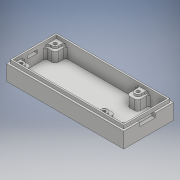
# Autodesk Inventor part: bottom
Saved by Autodesk Inventor 2018 (Build 220112000, 112)
## iProperties
Created: 2018-01-10
Part Number: bottom
Material: Generic
Document SubType Name: Modeling
Designer: gregg
Density: 1 g/cm^3
Appearance: Default
Author: gregg
Autodesk Inventor part; units mm, degrees
ref_plane "YZ Plane" through (0, 0, 0) normal (1, 0, 0) x (0, 1, 0)
ref_plane "XZ Plane" through (0, 0, 0) normal (0, 1, 0) x (-1, 0, 0)
ref_plane "XY Plane" through (0, 0, 0) normal (0, 0, 1) x (1, 0, 0)
sketch "Sketch1" plane through (0, 0, 0) normal (0, 0, 1) x (1, 0, 0)
  line L0 (0, 0) -> (100, 0)
  line L1 (100, 0) -> (100, 39)
  line L2 (100, 39) -> (0, 39)
  line L3 (0, 39) -> (0, 0)
  dimension "d46" = 39
  dimension "d47" = 100
  constraints: 8 end point, 2 parallel, 1 horizontal, 1 perpendicular
  measures "d46" distance between parallel lines of L0 L2
  measures "d47" distance between parallel lines of L1 L3
extrude "bottom" add sketch "Sketch1" along normal blind 3
sketch "Sketch5" plane through (0, 0, 0) normal (0, 0, -1) x (-1, 0, 0)
  line L0 (0, 0) -> (-100, 0) projected
  line L1 (0, 39) -> (0, 0) projected
  line L2 (-100, 39) -> (0, 39) projected
  line L3 (-100, 0) -> (-100, 39) projected
  line L4 (3, 42) -> (3, -3)
  line L5 (3, -3) -> (-103, -3)
  line L6 (-103, -3) -> (-103, 42)
  line L7 (-103, 42) -> (3, 42)
  dimension "d30" = 3
  constraints: 8 end point, 3 other
  measures "d30" distance between parallel lines of L2 L7
extrude "walls" add sketch "Sketch5" against normal blind 14
sketch "holes" plane through (0, 0, 3) normal (0, 0, 1) x (1, 0, 0)
  line L0 (0, 0) -> (100, 0) projected
  line L1 (100, 0) -> (100, 39) projected
  line L2 (100, 39) -> (0, 39) projected
  line L3 (0, 39) -> (0, 0) projected
  circle A0 centre (3.5, 34.5) radius 1.55 construction
  circle A1 centre (78.5, 34.5) radius 1.55 construction
  circle A2 centre (78.5, 3.5) radius 1.55 construction
  circle A3 centre (3.5, 3.5) radius 1.55 construction
  line L4 (3.5, 34.5) -> (3.5, 3.5) construction
  line L5 (3.5, 3.5) -> (78.5, 3.5) construction
  line L6 (78.5, 3.5) -> (78.5, 34.5) construction
  line L7 (78.5, 34.5) -> (3.5, 34.5) construction
  dimension "d33" = 3.1
  dimension "d34" = 75
  dimension "d35" = 31
  dimension "d58" = 3.5
  dimension "d59" = 3.5
  constraints: 8 end point, 4 centre point, 3 equal radius, 2 horizontal, 2 vertical
  measures "d33" diameter of A0
  measures "d34" distance of L6.end L4.start
  measures "d35" distance of L4.end L4.start
  measures "d58" distance from line of L4.end L3
  measures "d59" distance from line of L0 L4.end
sketch "Sketch8" plane through (103, -3, 0) normal (1, 0, 0) x (0, 0, -1)
  line L0 (-10.5, 14.297) -> (-14, 14.297)
  line L1 (-14, 14.297) -> (-14, 28.297)
  line L2 (-14, 28.297) -> (-10.5, 28.297)
  line L3 (-10.5, 28.297) -> (-10.5, 14.297)
  line L4 (-14, 0) -> (-14, 45) projected
  line L5 (-14, 28.297) -> (-10.5, 14.297) construction
  line L6 (-10.5, 28.297) -> (-14, 14.297) construction
  point P0 (0, 3)
  point P1 (-3, 37.5)
  point P2 (-3, 6.5)
  point P3 (-12.25, 21.297)
  dimension "d50" = 3.5
  dimension "d108" = 14.797
  dimension "d109" = 14
  constraints: 12 end point, 2 parallel, 1 horizontal, 1 midpoint, 1 perpendicular, 1 point on line
  measures "d50" distance of L1.end L2.end
  measures "d108" vertical distance of point (-3, 6.5) point (-12.25, 21.297)
  measures "d109" distance of L0.end L1.end
extrude "tip" cut sketch "Sketch8" against normal up to surface (3 mm away)
sketch "Sketch9" plane through (-3, -3, 0) normal (-1, 0, 0) x (0, 0, 1)
  line L0 (14, 16.412) -> (11, 16.412)
  line L1 (11, 16.412) -> (11, 24.912)
  line L2 (11, 24.912) -> (14, 24.912)
  line L3 (14, 24.912) -> (14, 16.412)
  line L4 (14, 45) -> (14, 0) projected
  line L5 (14, 25.5761) -> (11, 16.412) construction
  line L6 (14, 16.412) -> (11, 24.912) construction
  point P0 (0, 3)
  point P1 (3, 6.5)
  point P2 (3, 37.5)
  point P3 (3, 37.5)
  point P4 (3, 37.5)
  point P5 (12.5, 20.662)
  dimension "d53" = 3
  dimension "d110" = 14.162
  dimension "d111" = 8.5
  constraints: 12 end point, 2 parallel, 2 point on line, 1 horizontal, 1 midpoint, 1 perpendicular
  measures "d53" distance of L0.start L0.end
  measures "d110" vertical distance of point (3, 6.5) point (12.5, 20.662)
  measures "d111" distance of L2.end L0.start
extrude "uart" cut sketch "Sketch9" against normal up to surface (3 mm away)
sketch "Sketch7" plane through (0, 0, 3) normal (0, 0, 1) x (1, 0, 0)
  circle A0 centre (3.5, 34.5) radius 1.55 construction
  circle A1 centre (3.5, 3.5) radius 1.55 construction
  circle A2 centre (78.5, 3.5) radius 1.55 construction
  circle A3 centre (78.5, 34.5) radius 1.55 construction
  line L0 (0, 39) -> (0, 0) projected
  line L1 (2, 29.5) -> (8.5, 29.5)
  line L2 (8.5, 29.5) -> (8.5, 37)
  line L3 (100, 39) -> (0, 39) projected
  arc A4 (10.5, 39) -> (8.5, 37) centre (10.5, 37) ccw
  line L4 (0, 39) -> (100, 39) projected
  arc A5 (5.4, 29.5) -> (8.5, 32.6) centre (5.4, 32.6) ccw
  arc A6 (2, 29.5) -> (0, 27.5) centre (2, 27.5) ccw
  line L5 (0, 0) -> (0, 39) projected
  line L6 (1.7924, 37.3805) -> (5.1408, 37.4191)
  line L7 (5.1408, 37.4191) -> (6.8484, 34.5385)
  line L8 (6.8484, 34.5385) -> (5.2076, 31.6195)
  line L9 (5.2076, 31.6195) -> (1.8592, 31.5809)
  line L10 (1.8592, 31.5809) -> (0.1516, 34.4615)
  line L11 (0.1516, 34.4615) -> (1.7924, 37.3805)
  line L12 (100, 0) -> (0, 0) projected
  line L13 (0, 0) -> (0, 10.5)
  arc A7 (0, 10.5) -> (2, 8.5) centre (2, 10.5) ccw
  line L14 (2, 8.5) -> (5.4, 8.5)
  arc A8 (8.5, 5.4) -> (5.4, 8.5) centre (5.4, 5.4) ccw
  line L15 (8.5, 5.4) -> (8.5, 2)
  arc A9 (8.5, 2) -> (10.5, 0) centre (10.5, 2) ccw
  line L16 (10.5, 0) -> (0, 0)
  line L17 (85.5, 39) -> (71.5, 39)
  arc A10 (73.5, 37) -> (71.5, 39) centre (71.5, 37) ccw
  line L18 (73.5, 37) -> (73.5, 32.0359)
  line L19 (83.5, 32.0359) -> (83.5, 37)
  arc A11 (85.5, 39) -> (83.5, 37) centre (85.5, 37) ccw
  line L20 (71.5, 0) -> (85.5, 0)
  line L21 (0, 0) -> (100, 0) projected
  arc A12 (83.5, 2) -> (85.5, 0) centre (85.5, 2) ccw
  line L22 (83.5, 2) -> (83.5, 5.9641)
  line L23 (73.5, 5.9641) -> (73.5, 2)
  arc A13 (71.5, 0) -> (73.5, 2) centre (71.5, 2) ccw
  arc A14 (76.5, 8.9641) -> (73.5, 5.9641) centre (76.5, 5.9641) ccw
  line L24 (76.5, 8.9641) -> (80.5, 8.9641)
  arc A15 (83.5, 5.9641) -> (80.5, 8.9641) centre (80.5, 5.9641) ccw
  arc A16 (73.5, 32.0359) -> (76.5, 29.0359) centre (76.5, 32.0359) ccw
  arc A17 (80.5, 29.0359) -> (83.5, 32.0359) centre (80.5, 32.0359) ccw
  line L25 (76.5, 29.0359) -> (80.5, 29.0359)
  line L26 (75.5, 1.7679) -> (75.5, 5.2321) construction
  line L27 (75.5, 5.2321) -> (78.5, 6.9641) construction
  line L28 (78.5, 6.9641) -> (81.5, 5.2321) construction
  line L29 (81.5, 5.2321) -> (81.5, 1.7679) construction
  line L30 (81.5, 1.7679) -> (78.5, 0.0359) construction
  line L31 (78.5, 0.0359) -> (75.5, 1.7679) construction
  line L32 (78.5, 31.0359) -> (75.5, 32.7679) construction
  line L33 (75.5, 32.7679) -> (75.5, 36.2321) construction
  line L34 (75.5, 36.2321) -> (78.5, 37.9641) construction
  line L35 (78.5, 37.9641) -> (81.5, 36.2321) construction
  line L36 (81.5, 36.2321) -> (81.5, 32.7679) construction
  line L37 (81.5, 32.7679) -> (78.5, 31.0359) construction
  line L38 (78.5, 34.5) -> (73.5, 34.5) construction
  line L39 (78.5, 34.5) -> (83.5, 34.5) construction
  point P0 (78.5, 29.5)
  point P1 (78.5, 29.5)
  point P2 (78.5, 18.273)
  point P3 (78.5, 18.273)
  dimension "d38" = 5
  dimension "d39" = 5
  dimension "d40" = 2
  dimension "d41" = 3.1
  dimension "d42" = 2
  dimension "d60" = 5.8
  dimension "d77" = 5
  dimension "d78" = 5
  dimension "d79" = 3.1
  dimension "d87" = 6
  dimension "d88" = 10
  dimension "d89" = 2
  dimension "d90" = 3
  dimension "d91" = 6
  dimension "d92" = 2
  constraints: 68 end point, 28 point on circle, 28 tangent, 14 centre point, 12 point on line, 9 equal radius, 7 vertical, 5 coincident, 5 horizontal, 3 collinear, 3 perpendicular, 43 other
  measures "d38" distance from line of L2 A0.centre
  measures "d39" distance from line of L1 A0.centre
  measures "d40" radius of A4
  measures "d41" radius of A5
  measures "d42" radius of A6
  measures "d60" distance between parallel lines of L9 L6
  measures "d77" distance from line of L14 A1.centre
  measures "d78" distance from line of L15 A1.centre
  measures "d79" radius of A8
  measures "d87" distance between parallel lines of L26 L29
  measures "d88" distance between parallel lines of L22 L23
  measures "d89" distance from line of L24 L27.end
  measures "d90" radius of A15
  measures "d91" distance between parallel lines of L36 L33
  measures "d92" distance from line of L25 L32.start
extrude "standoffs" add sketch "Sketch7" along normal blind 9 contours L3 A4 L2 A5 L1 A6 L0 | L3 A11 L19 A17 L25 A16 L18 A10 | A13 L23 A14 L24 A15 L22 A12 L12 | A7 L14 A8 L15 A9 L12 L0 | L6 L7 L8 L9 L10 L11
sketch "Sketch10" plane through (0, 0, 12) normal (0, 0, 1) x (1, 0, 0)
  line L0 (2, 31.5) -> (3.4, 31.5)
  arc A0 (3.4, 31.5) -> (6.5, 34.6) centre (3.4, 34.6) ccw
  line L1 (6.5, 34.6) -> (6.5, 37)
  arc A1 (8.5, 39) -> (6.5, 37) centre (8.5, 37) ccw
  line L2 (8.5, 39) -> (0, 39)
  line L3 (0, 39) -> (0, 29.5)
  arc A2 (2, 29.5) -> (0, 27.5) centre (2, 27.5) ccw projected
  line L4 (2, 29.5) -> (5.4, 29.5) projected
  arc A3 (5.4, 29.5) -> (8.5, 32.6) centre (5.4, 32.6) ccw projected
  line L5 (8.5, 32.6) -> (8.5, 37) projected
  arc A4 (10.5, 39) -> (8.5, 37) centre (10.5, 37) ccw projected
  line L6 (0, 39) -> (10.5, 39) projected
  line L7 (0, 27.5) -> (0, 39) projected
  arc A5 (2, 31.5) -> (0, 29.5) centre (2, 29.5) ccw
  line L8 (3.5, 34.5) -> (3.5, 3.5) construction
  line L9 (78.5, 34.5) -> (3.5, 34.5) construction
  line L10 (0, 0) -> (0, 8.5)
  arc A6 (0, 8.5) -> (2, 6.5) centre (2, 8.5) ccw
  line L11 (2, 6.5) -> (3.4, 6.5)
  arc A7 (6.5, 3.4) -> (3.4, 6.5) centre (3.4, 3.4) ccw
  line L12 (6.5, 3.4) -> (6.5, 2)
  arc A8 (6.5, 2) -> (8.5, 0) centre (8.5, 2) ccw
  line L13 (8.5, 0) -> (0, 0)
  line L14 (100, 0) -> (0, 0) projected
  line L15 (78.5, 3.5) -> (78.5, 34.5) construction
  line L16 (3.5, 3.5) -> (78.5, 3.5) construction
  line L17 (71.5, 39) -> (85.5, 39) projected
  line L18 (73.5, 39) -> (83.5, 39)
  arc A9 (83.5, 39) -> (81.5, 37) centre (83.5, 37) ccw
  line L19 (81.5, 37) -> (81.5, 34.5)
  line L20 (75.5, 34.5) -> (75.5, 37)
  arc A10 (75.5, 37) -> (73.5, 39) centre (73.5, 37) ccw
  line L21 (0, 39) -> (100, 39) projected
  arc A11 (75.5, 34.5) -> (81.5, 34.5) centre (78.5, 34.5) ccw
  arc A12 (81.5, 3.5) -> (75.5, 3.5) centre (78.5, 3.5) ccw
  line L22 (81.5, 3.5) -> (81.5, 2)
  arc A13 (81.5, 2) -> (83.5, 0) centre (83.5, 2) ccw
  line L23 (83.5, 0) -> (73.5, 0)
  arc A14 (73.5, 0) -> (75.5, 2) centre (73.5, 2) ccw
  line L24 (75.5, 2) -> (75.5, 3.5)
  dimension "d61" = 3
  dimension "d62" = 3
  dimension "d63" = 2
  dimension "d64" = 3.1
  dimension "d65" = 2
  dimension "d80" = 3
  dimension "d81" = 3
  dimension "d96" = 6
  dimension "d97" = 6
  constraints: 28 end point, 25 tangent, 24 point on circle, 12 centre point, 7 equal radius, 6 point on line, 6 vertical, 3 perpendicular, 2 coincident, 1 horizontal
  measures "d61" distance from line of L0 L8.start
  measures "d62" distance from line of L1 L8.start
  measures "d63" radius of A1
  measures "d64" radius of A0
  measures "d65" radius of A5
  measures "d80" distance from line of L11 L8.end
  measures "d81" distance from line of L12 L8.end
  measures "d96" diameter of A11
  measures "d97" diameter of A12
extrude "finalStandoff" add sketch "Sketch10" along normal up to surface (2 mm away) contours A5 L3 L2 A1 L1 A0 L0 | L17 A9 L19 A11 L20 A10 | A14 L24 A12 L22 A13 L14 | L10 A6 L11 A7 L12 A8 L13
sketch "Sketch11" plane through (0, 0, 0) normal (0, 0, -1) x (-1, 0, 0)
  line L0 (-78.5, 34.5) -> (-3.5, 34.5) construction
  line L1 (-3.5, 34.5) -> (-3.5, 3.5) construction
  line L2 (-2.6034, 31.1539) -> (-5.9495, 32.0505)
  line L3 (-5.9495, 32.0505) -> (-6.8461, 35.3966)
  line L4 (-6.8461, 35.3966) -> (-4.3966, 37.8461)
  line L5 (-4.3966, 37.8461) -> (-1.0505, 36.9495)
  line L6 (-1.0505, 36.9495) -> (-0.1539, 33.6034)
  line L7 (-0.1539, 33.6034) -> (-2.6034, 31.1539)
  line L8 (-5.9495, 32.0505) -> (-3.5, 34.5) construction
  line L9 (-5.9495, 5.9495) -> (-2.6034, 6.8461)
  line L10 (-2.6034, 6.8461) -> (-0.1539, 4.3966)
  line L11 (-0.1539, 4.3966) -> (-1.0505, 1.0505)
  line L12 (-1.0505, 1.0505) -> (-4.3966, 0.1539)
  line L13 (-4.3966, 0.1539) -> (-6.8461, 2.6034)
  line L14 (-6.8461, 2.6034) -> (-5.9495, 5.9495)
  line L15 (-5.9495, 32.0505) -> (-5.9495, 5.9495) construction
  line L16 (-78.5, 3.5) -> (-78.5, 34.5) construction
  line L17 (-3.5, 3.5) -> (-78.5, 3.5) construction
  line L18 (-78.5, 31.0359) -> (-81.5, 32.7679)
  line L19 (-81.5, 32.7679) -> (-81.5, 36.2321)
  line L20 (-81.5, 36.2321) -> (-78.5, 37.9641)
  line L21 (-78.5, 37.9641) -> (-75.5, 36.2321)
  line L22 (-75.5, 36.2321) -> (-75.5, 32.7679)
  line L23 (-75.5, 32.7679) -> (-78.5, 31.0359)
  line L24 (-75.5, 5.2321) -> (-75.5, 1.7679)
  line L25 (-75.5, 1.7679) -> (-78.5, 0.0359)
  line L26 (-78.5, 0.0359) -> (-81.5, 1.7679)
  line L27 (-81.5, 1.7679) -> (-81.5, 5.2321)
  line L28 (-81.5, 5.2321) -> (-78.5, 6.9641)
  line L29 (-78.5, 6.9641) -> (-75.5, 5.2321)
  point P0 (0, 0)
  dimension "d68" = 6
  dimension "d69" = 45
  constraints: 52 end point, 4 coincident, 3 equal length, 3 vertical, 52 other
  measures "d68" distance between parallel lines of L4 L7
  measures "d69" angle of L0 L8
extrude "forNuts" cut sketch "Sketch11" against normal up to surface (12 mm away)
sketch "Sketch13" plane through (0, 0, 0) normal (0, 0, -1) x (-1, 0, 0)
  circle A0 centre (-3.5, 34.5) radius 1.55
  circle A1 centre (-3.5, 3.5) radius 1.55 projected
  circle A2 centre (-78.5, 34.5) radius 1.55 projected
  circle A3 centre (-78.5, 3.5) radius 1.55 projected
  point P0 (0, 0)
  dimension "d74" = 3.1
  constraints: 1 centre point, 1 coincident
  measures "d74" diameter of A0
extrude "mountHoles" cut sketch "Sketch13" along normal through all both and the other way through all
sketch "Sketch12" plane through (3.4, 31.5, 12) normal (0, 0, -1) x (-1, 0, 0)
  line L0 (-3.4461, 3.8966) -> (-0.9966, 6.3461) projected
  line L1 (-0.9966, 6.3461) -> (2.3495, 5.4495) projected
  line L2 (2.3495, 5.4495) -> (3.2461, 2.1034) projected
  line L3 (3.2461, 2.1034) -> (0.7966, -0.3461) projected
  line L4 (0.7966, -0.3461) -> (-2.5495, 0.5505) projected
  line L5 (-2.5495, 0.5505) -> (-3.4461, 3.8966) projected
  line L6 (2.3495, -30.4495) -> (-0.9966, -31.3461) projected
  line L7 (-0.9966, -31.3461) -> (-3.4461, -28.8966) projected
  line L8 (-3.4461, -28.8966) -> (-2.5495, -25.5505) projected
  line L9 (-2.5495, -25.5505) -> (0.7966, -24.6539) projected
  line L10 (0.7966, -24.6539) -> (3.2461, -27.1034) projected
  line L11 (3.2461, -27.1034) -> (2.3495, -30.4495) projected
  line L12 (6.4, 10.5) -> (6.4, -34.5) projected
  line L13 (-99.6, 10.5) -> (6.4, 10.5) projected
  line L14 (-99.6, -34.5) -> (-99.6, 10.5) projected
  line L15 (6.4, -34.5) -> (-99.6, -34.5) projected
  line L16 (-78.1, 4.7321) -> (-75.1, 6.4641) projected
  line L17 (-75.1, 6.4641) -> (-72.1, 4.7321) projected
  line L18 (-72.1, 4.7321) -> (-72.1, 1.2679) projected
  line L19 (-72.1, 1.2679) -> (-75.1, -0.4641) projected
  line L20 (-75.1, -0.4641) -> (-78.1, 1.2679) projected
  line L21 (-78.1, 1.2679) -> (-78.1, 4.7321) projected
  line L22 (-78.1, -29.7321) -> (-78.1, -26.2679) projected
  line L23 (-78.1, -26.2679) -> (-75.1, -24.5359) projected
  line L24 (-75.1, -24.5359) -> (-72.1, -26.2679) projected
  line L25 (-72.1, -26.2679) -> (-72.1, -29.7321) projected
  line L26 (-72.1, -29.7321) -> (-75.1, -31.4641) projected
  line L27 (-75.1, -31.4641) -> (-78.1, -29.7321) projected
  line L28 (3.2461, -27.1034) -> (2.3495, -30.4495) projected
  line L29 (2.3495, -30.4495) -> (-0.9966, -31.3461) projected
  line L30 (-0.9966, -31.3461) -> (-3.4461, -28.8966) projected
  line L31 (-3.4461, -28.8966) -> (-2.5495, -25.5505) projected
  line L32 (-2.5495, -25.5505) -> (0.7966, -24.6539) projected
  line L33 (0.7966, -24.6539) -> (3.2461, -27.1034) projected
  line L34 (-0.9966, 6.3461) -> (2.3495, 5.4495) projected
  line L35 (2.3495, 5.4495) -> (3.2461, 2.1034) projected
  line L36 (3.2461, 2.1034) -> (0.7966, -0.3461) projected
  line L37 (0.7966, -0.3461) -> (-2.5495, 0.5505) projected
  line L38 (-2.5495, 0.5505) -> (-3.4461, 3.8966) projected
  line L39 (-3.4461, 3.8966) -> (-0.9966, 6.3461) projected
  line L40 (6.4, 10.5) -> (6.4, -34.5) projected
  line L41 (-99.6, 10.5) -> (6.4, 10.5) projected
  line L42 (-99.6, -34.5) -> (-99.6, 10.5) projected
  line L43 (6.4, -34.5) -> (-99.6, -34.5) projected
extrude "fillBeforeHoles" add sketch "Sketch12" along normal blind 0.6 contours L0 L1 L2 L3 L4 L5 | L6 L7 L8 L9 L10 L11 | L16 L17 L18 L19 L20 L21 | L22 L23 L24 L25 L26 L27
sketch "Sketch14" plane through (0, 0, 3) normal (0, 0, 1) x (1, 0, 0)
  line L0 (21.673, 4.45) -> (35.673, 4.45)
  line L1 (35.673, 4.45) -> (35.673, 0.95)
  line L2 (35.673, 0.95) -> (21.673, 0.95)
  line L3 (21.673, 0.95) -> (21.673, 4.45)
  line L4 (3.5, 34.5) -> (3.5, 3.5) construction
  line L5 (3.5, 3.5) -> (78.5, 3.5) construction
  line L6 (21.673, 4.45) -> (35.673, 0.95) construction
  line L7 (35.673, 4.45) -> (21.673, 0.95) construction
  point P0 (0, 0)
  point P1 (28.673, 2.7)
  dimension "d112" = 25.173
  dimension "d113" = 0.8
  dimension "d114" = 3.5
  dimension "d115" = 14
  constraints: 12 end point, 2 parallel, 1 horizontal, 1 midpoint, 1 perpendicular
  measures "d112" horizontal distance of point (28.673, 2.7) L4.end
  measures "d113" vertical distance of point (28.673, 2.7) L4.end
  measures "d114" distance of L2.end L0.start
  measures "d115" distance of L1.end L2.end
extrude "jtag" cut sketch "Sketch14" along normal through all both and the other way through all
sketch "Sketch21" plane through (0, 0, 3) normal (0, 0, 1) x (1, 0, 0)
  circle A0 centre (91.75, 6.5) radius 7
  line L0 (83.5, 2) -> (83.5, 5.9641) projected
  line L1 (83.5, 6.5) -> (91.75, 6.5) construction
  line L2 (91.75, 6.5) -> (100, 6.5) construction
  line L3 (100, 0) -> (83.5, 0) projected
  line L4 (100, 11.297) -> (100, 0) projected
  arc A1 (83.5, 5.9641) -> (80.5, 8.9641) centre (80.5, 5.9641) ccw projected
  arc A2 (80.5, 8.9641) -> (86.8946, 11.5424) centre (80.5, 18.1833) ccw
  line L5 (80.5, 8.9641) -> (76.5, 8.9641) projected
  line L6 (100, 11.297) -> (100, 25.297) projected
  arc A3 (97.4895, 10.5073) -> (100, 11.297) centre (98.6205, 11.297) ccw
  arc A4 (83.5, 2) -> (85.5, 0) centre (85.5, 2) ccw projected
  line L7 (85.5, 0) -> (89.1519, 0)
  line L8 (85.5, 0) -> (100, 0) projected
  line L9 (94.3481, 0) -> (100, 0)
  point P0 (0, 0)
  dimension "d134" = 14
  dimension "d135" = 6.5
  constraints: 8 end point, 8 point on circle, 4 point on line, 4 tangent, 3 centre point, 2 collinear, 1 horizontal, 1 perpendicular
  measures "d134" diameter of A0
  measures "d135" distance from line of L3 L1.end
extrude "Extrusion21" add sketch "Sketch21" along normal blind 2.7
sketch "Sketch15" plane through (0, 0, 3) normal (0, 0, 1) x (1, 0, 0)
  circle A0 centre (91.75, 6.5) radius 4
  line L0 (35.673, 4.45) -> (35.673, 0.95) construction
  line L1 (35.673, 0.95) -> (21.673, 0.95) construction
  line L2 (21.673, 0.95) -> (21.673, 4.45) construction
  line L3 (21.673, 4.45) -> (35.673, 4.45) construction
  arc A1 (71.5, 0) -> (73.5, 2) centre (71.5, 2) ccw construction
  line L4 (73.5, 2) -> (73.5, 5.9641) construction
  arc A2 (76.5, 8.9641) -> (73.5, 5.9641) centre (76.5, 5.9641) ccw construction
  line L5 (76.5, 8.9641) -> (80.5, 8.9641) construction
  line L6 (100, 11.297) -> (100, 39) construction
  line L7 (100, 39) -> (85.5, 39) construction
  arc A3 (85.5, 39) -> (83.5, 37) centre (85.5, 37) ccw construction
  line L8 (83.5, 37) -> (83.5, 32.0359) construction
  arc A4 (80.5, 29.0359) -> (83.5, 32.0359) centre (80.5, 32.0359) ccw construction
  line L9 (80.5, 29.0359) -> (76.5, 29.0359) construction
  arc A5 (73.5, 32.0359) -> (76.5, 29.0359) centre (76.5, 32.0359) ccw construction
  line L10 (73.5, 32.0359) -> (73.5, 37) construction
  arc A6 (73.5, 37) -> (71.5, 39) centre (71.5, 37) ccw construction
  line L11 (71.5, 39) -> (10.5, 39) construction
  arc A7 (10.5, 39) -> (8.5, 37) centre (10.5, 37) ccw construction
  line L12 (8.5, 37) -> (8.5, 32.6) construction
  arc A8 (5.4, 29.5) -> (8.5, 32.6) centre (5.4, 32.6) ccw construction
  line L13 (5.4, 29.5) -> (2, 29.5) construction
  arc A9 (2, 29.5) -> (0, 27.5) centre (2, 27.5) ccw construction
  line L14 (0, 27.5) -> (0, 10.5) construction
  arc A10 (0, 10.5) -> (2, 8.5) centre (2, 10.5) ccw construction
  line L15 (2, 8.5) -> (5.4, 8.5) construction
  arc A11 (8.5, 5.4) -> (5.4, 8.5) centre (5.4, 5.4) ccw construction
  line L16 (8.5, 5.4) -> (8.5, 2) construction
  arc A12 (8.5, 2) -> (10.5, 0) centre (10.5, 2) ccw construction
  line L17 (10.5, 0) -> (71.5, 0) construction
  line L18 (91.75, 6.5) -> (83.5, 6.5) construction
  line L19 (91.75, 6.5) -> (100, 6.5) construction
  circle A13 centre (91.75, 6.5) radius 4.5 construction
  line L20 (84.8812, 11) -> (104.9849, 11) construction
  circle A14 centre (91.75, 6.5) radius 5.5 construction
  arc A15 (97.4895, 10.5073) -> (86.8946, 11.5424) centre (91.75, 6.5) ccw projected
  arc A16 (80.5, 8.9641) -> (86.8946, 11.5424) centre (80.5, 18.1833) ccw projected
  arc A17 (97.4895, 10.5073) -> (100, 11.297) centre (98.6205, 11.297) ccw projected
  point P0 (0, 0)
  dimension "d104" = 8
  dimension "d116" = 9
  dimension "d117" = 11
  constraints: 6 end point, 3 centre point, 2 coincident, 2 horizontal, 1 collinear, 1 point on line, 1 tangent
  measures "d104" diameter of A0
  measures "d116" diameter of A13
  measures "d117" diameter of A14
extrude "power" cut sketch "Sketch15" along normal through all both and the other way through all
sketch "Sketch16" plane through (0, 0, 0) normal (0, 0, -1) x (-1, 0, 0)
  circle A0 centre (-91.75, 6.5) radius 4 projected
  line L0 (-88.7478, 11.7) -> (-85.7456, 6.5)
  line L1 (-85.7456, 6.5) -> (-88.7478, 1.3)
  line L2 (-88.7478, 1.3) -> (-94.7522, 1.3)
  line L3 (-94.7522, 1.3) -> (-97.7544, 6.5)
  line L4 (-97.7544, 6.5) -> (-94.7522, 11.7)
  line L5 (-94.7522, 11.7) -> (-88.7478, 11.7)
  point P0 (0, 0)
  dimension "d118" = 10.4
  constraints: 12 end point, 1 coincident, 1 horizontal, 13 other
  measures "d118" distance between parallel lines of L2 L5
extrude "powerNut" cut sketch "Sketch16" against normal blind 3.1
sketch "Sketch17" plane through (0, 0, 3.1) normal (0, 0, -1) x (-1, 0, 0)
  line L0 (-88.7478, 11.7) -> (-85.7456, 6.5) projected
  line L1 (-94.7522, 11.7) -> (-88.7478, 11.7) projected
  line L2 (-97.7544, 6.5) -> (-94.7522, 11.7) projected
  line L3 (-94.7522, 1.3) -> (-97.7544, 6.5) projected
  line L4 (-88.7478, 1.3) -> (-94.7522, 1.3) projected
  line L5 (-85.7456, 6.5) -> (-88.7478, 1.3) projected
  point P0 (0, 0)
extrude "fillBeforePowerNut" add sketch "Sketch17" along normal blind 0.6
sketch "Sketch18" plane through (0, 0, 0) normal (0, 0, -1) x (-1, 0, 0)
  line L0 (-8.5363, 30.1182) -> (10.4943, 30.1182) construction
  line L1 (10.4943, 30.1182) -> (10.4943, 25.4403) construction
  line L2 (10.4943, 25.4403) -> (-8.5363, 25.4403) construction
  line L3 (-8.5363, 25.4403) -> (-8.5363, 30.1182) construction
  line L4 (-9.0093, 21.9531) -> (10.0213, 21.9531) construction
  line L5 (10.0213, 21.9531) -> (10.0213, 17.2752) construction
  line L6 (10.0213, 17.2752) -> (-9.0093, 17.2752) construction
  line L7 (-9.0093, 17.2752) -> (-9.0093, 21.9531) construction
  line L8 (-14.7037, 9.2364) -> (-14.7037, 13.9143) construction
  line L9 (-14.7037, 13.9143) -> (4.3268, 13.9143) construction
  line L10 (4.3268, 13.9143) -> (4.3268, 9.2364) construction
  line L11 (4.3268, 9.2364) -> (-14.7037, 9.2364) construction
  line L12 (-45.6184, 12.2142) -> (-26.5878, 12.2142) construction
  line L13 (-26.5878, 12.2142) -> (-26.5878, 7.5363) construction
  line L14 (-26.5878, 7.5363) -> (-45.6184, 7.5363) construction
  line L15 (-45.6184, 7.5363) -> (-45.6184, 12.2142) construction
  line L16 (-40.2506, 5.3058) -> (-21.22, 5.3058) construction
  line L17 (-21.22, 5.3058) -> (-21.22, 0.6279) construction
  line L18 (-21.22, 0.6279) -> (-40.2506, 0.6279) construction
  line L19 (-40.2506, 0.6279) -> (-40.2506, 5.3058) construction
  line L20 (-101.9782, 14.4275) -> (-101.9782, 19.1054) construction
  line L21 (-101.9782, 19.1054) -> (-61.9534, 19.1054) construction
  line L22 (-61.9534, 19.1054) -> (-61.9534, 14.4275) construction
  line L23 (-61.9534, 14.4275) -> (-101.9782, 14.4275) construction
  line L24 (-6.4947, 24.0182) -> (-6.4947, 29.3964)
  line L25 (-6.4947, 29.3964) -> (-8.5412, 29.3964)
  line L26 (-8.5412, 29.3964) -> (-8.5412, 30.1182)
  line L27 (-8.5412, 30.1182) -> (-3.6375, 30.1182)
  line L28 (-3.6375, 30.1182) -> (-3.6375, 29.3964)
  line L29 (-3.6375, 29.3964) -> (-5.684, 29.3964)
  line L30 (-5.684, 29.3964) -> (-5.684, 24.0182)
  line L31 (-5.684, 24.0182) -> (-6.4947, 24.0182)
  line L32 (1.197, 24.0182) -> (0.2677, 24.0182)
  line L33 (0.2677, 24.0182) -> (-1.2153, 26.4503)
  line L34 (-1.2153, 26.4503) -> (-2.7279, 24.0182)
  line L35 (-2.7279, 24.0182) -> (-3.6029, 24.0182)
  line L36 (-3.6029, 24.0182) -> (-1.6602, 27.0731)
  line L37 (-1.6602, 27.0731) -> (-3.5436, 30.1182)
  line L38 (-3.5436, 30.1182) -> (-2.6142, 30.1182)
  line L39 (-2.6142, 30.1182) -> (-1.1609, 27.7306)
  line L40 (-1.1609, 27.7306) -> (0.3221, 30.1182)
  line L41 (0.3221, 30.1182) -> (1.197, 30.1182)
  line L42 (1.197, 30.1182) -> (-0.7111, 27.1127)
  line L43 (-0.7111, 27.1127) -> (1.197, 24.0182)
  spline S0 degree 2 poles (-43.3, 5.8967) (-43.9624, 5.8967) (-44.8917, 6.1736) (-45.302, 6.3713) knots 0 0 0 1 2 2 2
  line L44 (-45.302, 6.3713) -> (-45.302, 7.3896)
  line L45 (-45.302, 7.3896) -> (-45.2427, 7.3896)
  spline S1 degree 2 poles (-45.2427, 7.3896) (-44.8423, 7.0139) (-43.8289, 6.5987) (-43.3593, 6.5987) knots 0 0 0 1 2 2 2
  spline S2 degree 2 poles (-43.3593, 6.5987) (-42.687, 6.5987) (-41.9999, 7.1573) (-41.9999, 7.617) knots 0 0 0 1 2 2 2
  spline S3 degree 2 poles (-41.9999, 7.617) (-41.9999, 7.9828) (-42.3607, 8.4376) (-42.7513, 8.5513) knots 0 0 0 1 2 2 2
  spline S4 degree 2 poles (-42.7513, 8.5513) (-43.033, 8.6304) (-43.5026, 8.7391) (-43.8536, 8.8281) knots 0 0 0 1 2 2 2
  spline S5 degree 2 poles (-43.8536, 8.8281) (-44.17, 8.9121) (-44.6692, 9.1642) (-44.862, 9.3669) knots 0 0 0 1 2 2 2
  spline S6 degree 2 poles (-44.862, 9.3669) (-45.0499, 9.5696) (-45.2575, 10.1133) (-45.2575, 10.4693) knots 0 0 0 1 2 2 2
  spline S7 degree 2 poles (-45.2575, 10.4693) (-45.2575, 11.2108) (-44.1008, 12.2142) (-43.206, 12.2142) knots 0 0 0 1 2 2 2
  spline S8 degree 2 poles (-43.206, 12.2142) (-42.6919, 12.2142) (-41.7824, 12.0116) (-41.3919, 11.8188) knots 0 0 0 1 2 2 2
  line L46 (-41.3919, 11.8188) -> (-41.3919, 10.8499)
  line L47 (-41.3919, 10.8499) -> (-41.4512, 10.8499)
  spline S9 degree 2 poles (-41.4512, 10.8499) (-41.7428, 11.1168) (-42.6524, 11.5123) (-43.1517, 11.5123) knots 0 0 0 1 2 2 2
  spline S10 degree 2 poles (-43.1517, 11.5123) (-43.7152, 11.5123) (-44.4122, 10.9834) (-44.4122, 10.5533) knots 0 0 0 1 2 2 2
  spline S11 degree 2 poles (-44.4122, 10.5533) (-44.4122, 10.1677) (-44.0019, 9.708) (-43.6163, 9.6042) knots 0 0 0 1 2 2 2
  spline S12 degree 2 poles (-43.6163, 9.6042) (-43.3593, 9.535) (-42.6128, 9.357) (-42.3657, 9.2829) knots 0 0 0 1 2 2 2
  spline S13 degree 2 poles (-42.3657, 9.2829) (-41.7379, 9.0901) (-41.1546, 8.314) (-41.1546, 7.7455) knots 0 0 0 1 2 2 2
  spline S14 degree 2 poles (-41.1546, 7.7455) (-41.1546, 7.3847) (-41.4462, 6.6926) (-41.7082, 6.4504) knots 0 0 0 1 2 2 2
  spline S15 degree 2 poles (-41.7082, 6.4504) (-41.9999, 6.1834) (-42.7414, 5.8967) (-43.3, 5.8967) knots 0 0 0 1 2 2 2
  line L48 (-38.9054, 6.0055) -> (-38.9054, 11.3838)
  line L49 (-38.9054, 11.3838) -> (-40.9519, 11.3838)
  line L50 (-40.9519, 11.3838) -> (-40.9519, 12.1055)
  line L51 (-40.9519, 12.1055) -> (-36.0482, 12.1055)
  line L52 (-36.0482, 12.1055) -> (-36.0482, 11.3838)
  line L53 (-36.0482, 11.3838) -> (-38.0947, 11.3838)
  line L54 (-38.0947, 11.3838) -> (-38.0947, 6.0055)
  line L55 (-38.0947, 6.0055) -> (-38.9054, 6.0055)
  line L56 (-31.8958, 6.0055) -> (-35.4303, 6.0055)
  line L57 (-35.4303, 6.0055) -> (-35.4303, 12.1055)
  line L58 (-35.4303, 12.1055) -> (-34.6196, 12.1055)
  line L59 (-34.6196, 12.1055) -> (-34.6196, 6.7272)
  line L60 (-34.6196, 6.7272) -> (-31.8958, 6.7272)
  line L61 (-31.8958, 6.7272) -> (-31.8958, 6.0055)
  line L62 (-29.1325, 6.0055) -> (-31.4954, 6.0055)
  line L63 (-31.4954, 6.0055) -> (-31.4954, 6.6283)
  line L64 (-31.4954, 6.6283) -> (-30.7193, 6.6283)
  line L65 (-30.7193, 6.6283) -> (-30.7193, 11.4826)
  line L66 (-30.7193, 11.4826) -> (-31.4954, 11.4826)
  line L67 (-31.4954, 11.4826) -> (-31.4954, 12.1055)
  line L68 (-31.4954, 12.1055) -> (-29.1325, 12.1055)
  line L69 (-29.1325, 12.1055) -> (-29.1325, 11.4826)
  line L70 (-29.1325, 11.4826) -> (-29.9086, 11.4826)
  line L71 (-29.9086, 11.4826) -> (-29.9086, 6.6283)
  line L72 (-29.9086, 6.6283) -> (-29.1325, 6.6283)
  line L73 (-29.1325, 6.6283) -> (-29.1325, 6.0055)
  line L74 (-23.7641, 6.0055) -> (-24.6737, 6.0055)
  line L75 (-24.6737, 6.0055) -> (-27.3727, 11.2651)
  line L76 (-27.3727, 11.2651) -> (-27.3727, 6.0055)
  line L77 (-27.3727, 6.0055) -> (-28.129, 6.0055)
  line L78 (-28.129, 6.0055) -> (-28.129, 12.1055)
  line L79 (-28.129, 12.1055) -> (-26.9773, 12.1055)
  line L80 (-26.9773, 12.1055) -> (-24.5205, 7.2759)
  line L81 (-24.5205, 7.2759) -> (-24.5205, 12.1055)
  line L82 (-24.5205, 12.1055) -> (-23.7641, 12.1055)
  line L83 (-23.7641, 12.1055) -> (-23.7641, 6.0055)
  line L84 (-18.0794, 6.0055) -> (-19.1323, 6.0055)
  line L85 (-19.1323, 6.0055) -> (-21.3617, 8.8429)
  line L86 (-21.3617, 8.8429) -> (-21.7176, 8.4425)
  line L87 (-21.7176, 8.4425) -> (-21.7176, 6.0055)
  line L88 (-21.7176, 6.0055) -> (-22.5283, 6.0055)
  line L89 (-22.5283, 6.0055) -> (-22.5283, 12.1055)
  line L90 (-22.5283, 12.1055) -> (-21.7176, 12.1055)
  line L91 (-21.7176, 12.1055) -> (-21.7176, 9.3026)
  line L92 (-21.7176, 9.3026) -> (-19.2163, 12.1055)
  line L93 (-19.2163, 12.1055) -> (-18.2277, 12.1055)
  line L94 (-18.2277, 12.1055) -> (-20.7537, 9.3817)
  line L95 (-20.7537, 9.3817) -> (-18.0794, 6.0055)
  line L96 (-36.3503, -0.814) -> (-39.3262, -0.814)
  line L97 (-39.3262, -0.814) -> (-39.3262, -0.1911)
  line L98 (-39.3262, -0.1911) -> (-38.2189, -0.1911)
  line L99 (-38.2189, -0.1911) -> (-38.2189, 3.897)
  line L100 (-38.2189, 3.897) -> (-39.3262, 3.897)
  line L101 (-39.3262, 3.897) -> (-39.3262, 4.4556)
  spline S16 degree 2 poles (-39.3262, 4.4556) (-38.6984, 4.4556) (-38.1052, 4.8115) (-38.0656, 5.3058) knots 0 0 0 1 2 2 2
  line L102 (-38.0656, 5.3058) -> (-37.4329, 5.3058)
  line L103 (-37.4329, 5.3058) -> (-37.4329, -0.1911)
  line L104 (-37.4329, -0.1911) -> (-36.3503, -0.1911)
  line L105 (-36.3503, -0.1911) -> (-36.3503, -0.814)
  spline S17 degree 2 poles (-11.5302, 7.5869) (-12.1777, 7.5869) (-13.2504, 7.9824) (-13.636, 8.3828) knots 0 0 0 1 2 2 2
  spline S18 degree 2 poles (-13.636, 8.3828) (-14.0216, 8.7882) (-14.4319, 9.9844) (-14.4319, 10.7605) knots 0 0 0 1 2 2 2
  spline S19 degree 2 poles (-14.4319, 10.7605) (-14.4319, 11.4971) (-14.0166, 12.6637) (-13.631, 13.0789) knots 0 0 0 1 2 2 2
  spline S20 degree 2 poles (-13.631, 13.0789) (-13.2603, 13.4793) (-12.1728, 13.9143) (-11.5252, 13.9143) knots 0 0 0 1 2 2 2
  spline S21 degree 2 poles (-11.5252, 13.9143) (-11.2138, 13.9143) (-10.6503, 13.8254) (-10.3932, 13.7463) knots 0 0 0 1 2 2 2
  spline S22 degree 2 poles (-10.3932, 13.7463) (-10.1856, 13.6869) (-9.6814, 13.4694) (-9.5281, 13.3903) knots 0 0 0 1 2 2 2
  line L106 (-9.5281, 13.3903) -> (-9.5281, 12.4116)
  line L107 (-9.5281, 12.4116) -> (-9.5973, 12.4116)
  spline S23 degree 2 poles (-9.5973, 12.4116) (-9.7506, 12.545) (-10.0719, 12.7873) (-10.3685, 12.9257) knots 0 0 0 1 2 2 2
  spline S24 degree 2 poles (-10.3685, 12.9257) (-10.6156, 13.0493) (-11.2533, 13.2124) (-11.6191, 13.2124) knots 0 0 0 1 2 2 2
  spline S25 degree 2 poles (-11.6191, 13.2124) (-12.499, 13.2124) (-13.5866, 11.8876) (-13.5866, 10.7852) knots 0 0 0 1 2 2 2
  spline S26 degree 2 poles (-13.5866, 10.7852) (-13.5866, 10.1723) (-13.2998, 9.2528) (-13.028, 8.9365) knots 0 0 0 1 2 2 2
  spline S27 degree 2 poles (-13.028, 8.9365) (-12.766, 8.6201) (-12.0245, 8.2889) (-11.5598, 8.2889) knots 0 0 0 1 2 2 2
  spline S28 degree 2 poles (-11.5598, 8.2889) (-11.2187, 8.2889) (-10.5366, 8.3878) (-10.3042, 8.4866) knots 0 0 0 1 2 2 2
  line L108 (-10.3042, 8.4866) -> (-10.3042, 10.0635)
  line L109 (-10.3042, 10.0635) -> (-11.718, 10.0635)
  line L110 (-11.718, 10.0635) -> (-11.718, 10.7754)
  line L111 (-11.718, 10.7754) -> (-9.5034, 10.7754)
  line L112 (-9.5034, 10.7754) -> (-9.5034, 8.1109)
  spline S29 degree 2 poles (-9.5034, 8.1109) (-9.6567, 8.0417) (-10.1806, 7.8292) (-10.4031, 7.7649) knots 0 0 0 1 2 2 2
  spline S30 degree 2 poles (-10.4031, 7.7649) (-10.7046, 7.6759) (-11.1891, 7.5869) (-11.5302, 7.5869) knots 0 0 0 1 2 2 2
  line L113 (-4.1202, 7.7056) -> (-5.0298, 7.7056)
  line L114 (-5.0298, 7.7056) -> (-7.7288, 12.9652)
  line L115 (-7.7288, 12.9652) -> (-7.7288, 7.7056)
  line L116 (-7.7288, 7.7056) -> (-8.4851, 7.7056)
  line L117 (-8.4851, 7.7056) -> (-8.4851, 13.8056)
  line L118 (-8.4851, 13.8056) -> (-7.3333, 13.8056)
  line L119 (-7.3333, 13.8056) -> (-4.8765, 8.976)
  line L120 (-4.8765, 8.976) -> (-4.8765, 13.8056)
  line L121 (-4.8765, 13.8056) -> (-4.1202, 13.8056)
  line L122 (-4.1202, 13.8056) -> (-4.1202, 7.7056)
  spline S31 degree 2 poles (1.9254, 10.7506) (1.9254, 9.9152) (1.2482, 8.5707) (0.6797, 8.195) knots 0 0 0 1 2 2 2
  spline S32 degree 2 poles (0.6797, 8.195) (0.2151, 7.9033) (-0.739, 7.7056) (-1.4805, 7.7056) knots 0 0 0 1 2 2 2
  line L123 (-1.4805, 7.7056) -> (-2.8844, 7.7056)
  line L124 (-2.8844, 7.7056) -> (-2.8844, 13.8056)
  line L125 (-2.8844, 13.8056) -> (-1.4953, 13.8056)
  spline S33 degree 2 poles (-1.4953, 13.8056) (-0.6352, 13.8056) (0.3436, 13.5485) (0.6896, 13.3211) knots 0 0 0 1 2 2 2
  spline S34 degree 2 poles (0.6896, 13.3211) (1.2779, 12.9306) (1.9254, 11.6404) (1.9254, 10.7506) knots 0 0 0 1 2 2 2
  spline S35 degree 2 poles (1.0801, 10.7605) (1.0801, 11.4625) (0.6155, 12.4561) (0.1557, 12.7378) knots 0 0 0 1 2 2 2
  spline S36 degree 2 poles (0.1557, 12.7378) (-0.1705, 12.9306) (-0.9071, 13.1036) (-1.4558, 13.1036) knots 0 0 0 1 2 2 2
  line L126 (-1.4558, 13.1036) -> (-2.0737, 13.1036)
  line L127 (-2.0737, 13.1036) -> (-2.0737, 8.4075)
  line L128 (-2.0737, 8.4075) -> (-1.4558, 8.4075)
  spline S37 degree 2 poles (-1.4558, 8.4075) (-0.9169, 8.4075) (-0.1013, 8.5805) (0.2299, 8.8129) knots 0 0 0 1 2 2 2
  spline S38 degree 2 poles (0.2299, 8.8129) (0.655, 9.0996) (1.0801, 10.0487) (1.0801, 10.7605) knots 0 0 0 1 2 2 2
  line L129 (-3.6705, 15.8531) -> (-4.7234, 15.8531)
  line L130 (-4.7234, 15.8531) -> (-6.6513, 18.2802)
  line L131 (-6.6513, 18.2802) -> (-7.5807, 18.2802)
  line L132 (-7.5807, 18.2802) -> (-7.5807, 15.8531)
  line L133 (-7.5807, 15.8531) -> (-8.3913, 15.8531)
  line L134 (-8.3913, 15.8531) -> (-8.3913, 21.9531)
  line L135 (-8.3913, 21.9531) -> (-6.8194, 21.9531)
  spline S39 degree 2 poles (-6.8194, 21.9531) (-6.2954, 21.9531) (-5.5885, 21.8394) (-5.2672, 21.6318) knots 0 0 0 1 2 2 2
  spline S40 degree 2 poles (-5.2672, 21.6318) (-4.9459, 21.4241) (-4.5751, 20.7766) (-4.5751, 20.2971) knots 0 0 0 1 2 2 2
  spline S41 degree 2 poles (-4.5751, 20.2971) (-4.5751, 19.6297) (-5.2573, 18.7251) (-5.8406, 18.5076) knots 0 0 0 1 2 2 2
  line L136 (-5.8406, 18.5076) -> (-3.6705, 15.8531)
  spline S42 degree 2 poles (-5.4204, 20.2328) (-5.4204, 20.4997) (-5.6083, 20.91) (-5.806, 21.0435) knots 0 0 0 1 2 2 2
  spline S43 degree 2 poles (-5.806, 21.0435) (-5.979, 21.1572) (-6.4388, 21.2511) (-6.7749, 21.2511) knots 0 0 0 1 2 2 2
  line L137 (-6.7749, 21.2511) -> (-7.5807, 21.2511)
  line L138 (-7.5807, 21.2511) -> (-7.5807, 18.9574)
  line L139 (-7.5807, 18.9574) -> (-6.8688, 18.9574)
  spline S44 degree 2 poles (-6.8688, 18.9574) (-6.5178, 18.9574) (-5.9593, 19.081) (-5.7665, 19.2738) knots 0 0 0 1 2 2 2
  spline S45 degree 2 poles (-5.7665, 19.2738) (-5.5885, 19.4419) (-5.4204, 19.9164) (-5.4204, 20.2328) knots 0 0 0 1 2 2 2
  line L140 (1.0305, 15.8531) -> (0.1012, 15.8531)
  line L141 (0.1012, 15.8531) -> (-1.3818, 18.2852)
  line L142 (-1.3818, 18.2852) -> (-2.8944, 15.8531)
  line L143 (-2.8944, 15.8531) -> (-3.7694, 15.8531)
  line L144 (-3.7694, 15.8531) -> (-1.8267, 18.908)
  line L145 (-1.8267, 18.908) -> (-3.7101, 21.9531)
  line L146 (-3.7101, 21.9531) -> (-2.7807, 21.9531)
  line L147 (-2.7807, 21.9531) -> (-1.3274, 19.5655)
  line L148 (-1.3274, 19.5655) -> (0.1556, 21.9531)
  line L149 (0.1556, 21.9531) -> (1.0305, 21.9531)
  line L150 (1.0305, 21.9531) -> (-0.8776, 18.9476)
  line L151 (-0.8776, 18.9476) -> (1.0305, 15.8531)
  line L152 (-98.078, 12.8768) -> (-101.0538, 12.8768)
  line L153 (-101.0538, 12.8768) -> (-101.0538, 13.4997)
  line L154 (-101.0538, 13.4997) -> (-99.9465, 13.4997)
  line L155 (-99.9465, 13.4997) -> (-99.9465, 17.5878)
  line L156 (-99.9465, 17.5878) -> (-101.0538, 17.5878)
  line L157 (-101.0538, 17.5878) -> (-101.0538, 18.1464)
  spline S46 degree 2 poles (-101.0538, 18.1464) (-100.426, 18.1464) (-99.8328, 18.5023) (-99.7933, 18.9966) knots 0 0 0 1 2 2 2
  line L158 (-99.7933, 18.9966) -> (-99.1605, 18.9966)
  line L159 (-99.1605, 18.9966) -> (-99.1605, 13.4997)
  line L160 (-99.1605, 13.4997) -> (-98.078, 13.4997)
  line L161 (-98.078, 13.4997) -> (-98.078, 12.8768)
  line L162 (-93.194, 12.8768) -> (-96.9558, 12.8768)
  line L163 (-96.9558, 12.8768) -> (-96.9558, 13.7419)
  spline S47 degree 2 poles (-96.9558, 13.7419) (-96.5505, 14.1225) (-95.8288, 14.8294) (-95.4827, 15.2101) knots 0 0 0 1 2 2 2
  spline S48 degree 2 poles (-95.4827, 15.2101) (-94.7857, 15.9763) (-94.2766, 16.8957) (-94.2766, 17.3851) knots 0 0 0 1 2 2 2
  spline S49 degree 2 poles (-94.2766, 17.3851) (-94.2766, 17.6421) (-94.4348, 18.0277) (-94.5781, 18.1513) knots 0 0 0 1 2 2 2
  spline S50 degree 2 poles (-94.5781, 18.1513) (-94.7215, 18.2749) (-95.0972, 18.3985) (-95.3246, 18.3985) knots 0 0 0 1 2 2 2
  spline S51 degree 2 poles (-95.3246, 18.3985) (-95.5421, 18.3985) (-95.987, 18.2897) (-96.1896, 18.2057) knots 0 0 0 1 2 2 2
  spline S52 degree 2 poles (-96.1896, 18.2057) (-96.3626, 18.1365) (-96.684, 17.9387) (-96.7828, 17.8695) knots 0 0 0 1 2 2 2
  line L164 (-96.7828, 17.8695) -> (-96.8273, 17.8695)
  line L165 (-96.8273, 17.8695) -> (-96.8273, 18.7396)
  spline S53 degree 2 poles (-96.8273, 18.7396) (-96.5752, 18.8631) (-95.6706, 19.1054) (-95.2652, 19.1054) knots 0 0 0 1 2 2 2
  spline S54 degree 2 poles (-95.2652, 19.1054) (-94.4101, 19.1054) (-93.4461, 18.2007) (-93.4461, 17.4296) knots 0 0 0 1 2 2 2
  spline S55 degree 2 poles (-93.4461, 17.4296) (-93.4461, 17.0687) (-93.6142, 16.4656) (-93.7625, 16.2086) knots 0 0 0 1 2 2 2
  spline S56 degree 2 poles (-93.7625, 16.2086) (-93.9108, 15.9417) (-94.3408, 15.4177) (-94.5781, 15.1656) knots 0 0 0 1 2 2 2
  spline S57 degree 2 poles (-94.5781, 15.1656) (-94.9637, 14.7454) (-95.9079, 13.8457) (-96.1896, 13.5837) knots 0 0 0 1 2 2 2
  line L166 (-96.1896, 13.5837) -> (-93.194, 13.5837)
  line L167 (-93.194, 13.5837) -> (-93.194, 12.8768)
  line L168 (-85.1612, 18.9768) -> (-87.2621, 12.8768)
  line L169 (-87.2621, 12.8768) -> (-88.137, 12.8768)
  line L170 (-88.137, 12.8768) -> (-90.2379, 18.9768)
  line L171 (-90.2379, 18.9768) -> (-89.3679, 18.9768)
  line L172 (-89.3679, 18.9768) -> (-87.6773, 13.91)
  line L173 (-87.6773, 13.91) -> (-85.9867, 18.9768)
  line L174 (-85.9867, 18.9768) -> (-85.1612, 18.9768)
  spline S58 degree 2 poles (-77.1481, 15.9219) (-77.1481, 15.0865) (-77.8254, 13.7419) (-78.3938, 13.3662) knots 0 0 0 1 2 2 2
  spline S59 degree 2 poles (-78.3938, 13.3662) (-78.8585, 13.0746) (-79.8126, 12.8768) (-80.5541, 12.8768) knots 0 0 0 1 2 2 2
  line L175 (-80.5541, 12.8768) -> (-81.9579, 12.8768)
  line L176 (-81.9579, 12.8768) -> (-81.9579, 18.9768)
  line L177 (-81.9579, 18.9768) -> (-80.5689, 18.9768)
  spline S60 degree 2 poles (-80.5689, 18.9768) (-79.7088, 18.9768) (-78.73, 18.7198) (-78.384, 18.4924) knots 0 0 0 1 2 2 2
  spline S61 degree 2 poles (-78.384, 18.4924) (-77.7957, 18.1019) (-77.1481, 16.8117) (-77.1481, 15.9219) knots 0 0 0 1 2 2 2
  spline S62 degree 2 poles (-77.9934, 15.9318) (-77.9934, 16.6337) (-78.4581, 17.6273) (-78.9178, 17.9091) knots 0 0 0 1 2 2 2
  spline S63 degree 2 poles (-78.9178, 17.9091) (-79.2441, 18.1019) (-79.9806, 18.2749) (-80.5293, 18.2749) knots 0 0 0 1 2 2 2
  line L178 (-80.5293, 18.2749) -> (-81.1472, 18.2749)
  line L179 (-81.1472, 18.2749) -> (-81.1472, 13.5788)
  line L180 (-81.1472, 13.5788) -> (-80.5293, 13.5788)
  spline S64 degree 2 poles (-80.5293, 13.5788) (-79.9905, 13.5788) (-79.1749, 13.7518) (-78.8437, 13.9841) knots 0 0 0 1 2 2 2
  spline S65 degree 2 poles (-78.8437, 13.9841) (-78.4186, 14.2708) (-77.9934, 15.2199) (-77.9934, 15.9318) knots 0 0 0 1 2 2 2
  spline S66 degree 2 poles (-73.8856, 12.7681) (-74.4788, 12.7681) (-75.4823, 13.1685) (-75.8481, 13.5689) knots 0 0 0 1 2 2 2
  spline S67 degree 2 poles (-75.8481, 13.5689) (-76.2139, 13.9643) (-76.6143, 15.1507) (-76.6143, 15.9219) knots 0 0 0 1 2 2 2
  spline S68 degree 2 poles (-76.6143, 15.9219) (-76.6143, 16.6881) (-76.2237, 17.825) (-75.853, 18.2452) knots 0 0 0 1 2 2 2
  spline S69 degree 2 poles (-75.853, 18.2452) (-75.4872, 18.6555) (-74.4887, 19.0856) (-73.8707, 19.0856) knots 0 0 0 1 2 2 2
  spline S70 degree 2 poles (-73.8707, 19.0856) (-73.5643, 19.0856) (-73.0254, 18.9966) (-72.7981, 18.9274) knots 0 0 0 1 2 2 2
  spline S71 degree 2 poles (-72.7981, 18.9274) (-72.6003, 18.8631) (-72.19, 18.6802) (-71.9874, 18.5715) knots 0 0 0 1 2 2 2
  line L181 (-71.9874, 18.5715) -> (-71.9874, 17.5927)
  line L182 (-71.9874, 17.5927) -> (-72.0516, 17.5927)
  spline S72 degree 2 poles (-72.0516, 17.5927) (-72.1604, 17.6916) (-72.4965, 17.9684) (-72.7387, 18.1019) knots 0 0 0 1 2 2 2
  spline S73 degree 2 poles (-72.7387, 18.1019) (-72.9711, 18.2304) (-73.5198, 18.3935) (-73.8757, 18.3935) knots 0 0 0 1 2 2 2
  spline S74 degree 2 poles (-73.8757, 18.3935) (-74.2662, 18.3935) (-74.9632, 18.0722) (-75.2252, 17.7657) knots 0 0 0 1 2 2 2
  spline S75 degree 2 poles (-75.2252, 17.7657) (-75.4823, 17.4543) (-75.769, 16.5101) (-75.769, 15.9219) knots 0 0 0 1 2 2 2
  spline S76 degree 2 poles (-75.769, 15.9219) (-75.769, 15.2941) (-75.4674, 14.3895) (-75.2054, 14.078) knots 0 0 0 1 2 2 2
  spline S77 degree 2 poles (-75.2054, 14.078) (-74.9484, 13.7765) (-74.2613, 13.47) (-73.8757, 13.47) knots 0 0 0 1 2 2 2
  spline S78 degree 2 poles (-73.8757, 13.47) (-73.5247, 13.47) (-72.9266, 13.643) (-72.6943, 13.7716) knots 0 0 0 1 2 2 2
  spline S79 degree 2 poles (-72.6943, 13.7716) (-72.4718, 13.9001) (-72.1406, 14.167) (-72.0467, 14.2609) knots 0 0 0 1 2 2 2
  line L183 (-72.0467, 14.2609) -> (-71.9874, 14.2609)
  line L184 (-71.9874, 14.2609) -> (-71.9874, 13.2921)
  spline S80 degree 2 poles (-71.9874, 13.2921) (-72.19, 13.1981) (-72.546, 13.0251) (-72.7981, 12.946) knots 0 0 0 1 2 2 2
  spline S81 degree 2 poles (-72.7981, 12.946) (-73.065, 12.8571) (-73.5198, 12.7681) (-73.8856, 12.7681) knots 0 0 0 1 2 2 2
  point P0 (0, 0)
  constraints: 12 other
extrude "Text" cut sketch "Sketch18" against normal blind 0.7
sketch "Sketch19" plane through (0, 0, 14) normal (0, 0, 1) x (1, 0, 0)
  line L0 (0, 27.5) -> (0, 10.5) projected
  line L1 (0, 21.9123) -> (0, 39)
  line L2 (0, 39) -> (100, 39)
  line L3 (100, 11.297) -> (100, 25.297) projected
  line L4 (100, 39) -> (100, 0)
  line L5 (103, 25.297) -> (103, 42) construction
  line L6 (100, 39) -> (100, 25.297) construction
  line L7 (101.3, -1.3) -> (101.3, 40.3)
  line L8 (101.3, 40.3) -> (-1.3, 40.3)
  line L9 (-1.3, 40.3) -> (-1.3, -1.3)
  line L10 (-3, 21.912) -> (0, 21.912) projected
  line L11 (100, 39) -> (100, 40.3) construction
  line L12 (0, 39) -> (-1.3, 39) construction
  line L13 (103, 11.297) -> (100, 11.297) projected
  line L14 (101.3, -1.3) -> (-1.3, -1.3)
  line L15 (0, 13.412) -> (-3, 13.412) projected
  line L16 (0, 13.412) -> (0, 0)
  line L17 (100, 0) -> (83.5, 0) projected
  line L18 (0, 0) -> (100, 0)
  line L19 (100, 0) -> (100, -1.3) construction
  line L20 (100, 39) -> (101.3, 39) construction
  line L21 (0, 39) -> (0, 40.3) construction
  line L22 (0, 0) -> (-1.3, 0) construction
  line L23 (0, 0) -> (0, -1.3) construction
  point P0 (101.3, 11.297)
  point P1 (-1.869, 13.412)
  dimension "d125" = 3
  dimension "d130" = 1.3
  constraints: 33 end point, 11 point on line, 7 perpendicular, 6 vertical, 4 horizontal
  measures "d125" distance between parallel lines of L5 L6
  measures "d130" distance between parallel lines of L7 L3
extrude "collar" add sketch "Sketch19" along normal blind 3 contours L0 L10 L9 L8 L7 L13 L3 L4 L2 L1 | L0 L15 L9 L10 | L0 L16 L18 L17 L4 L13 L7 L14 L9 L15
body "Solid1"
